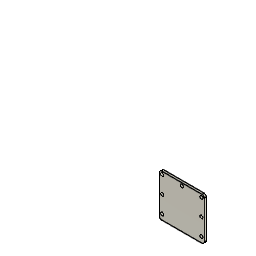
Power Panel Pro Compact - BLANK (Autodesk Fusion 360 design; units mm, degrees)
Autodesk Fusion 360 part; units mm, degrees
sketch "Sketch1" plane through (0, 175, 0) normal (0, 1, 0) x (-1, 0, 0)
  circle A0 centre (-78.5, 56) radius 1.95
  line L0 (86.5, 125) -> (-86.5, 125)
  line L1 (-86.5, 125) -> (-86.5, 0)
  line L2 (-86.5, 0) -> (86.5, 0)
  line L3 (86.5, 0) -> (86.5, 125)
  circle A1 centre (-78.5, 7.75) radius 1.95
  circle A2 centre (-23, 7.75) radius 1.95
  circle A3 centre (-11, 53.5) radius 1.95
  circle A4 centre (80.5, 53.5) radius 1.95
  circle A5 centre (80.5, 99.25) radius 1.95
  circle A6 centre (-23, 56) radius 1.95
  circle A7 centre (-50.75, 56) radius 1.95
  circle A8 centre (-78.5, 31.875) radius 1.95
  circle A9 centre (-11, 7.75) radius 1.95
  circle A10 centre (-11, 99.25) radius 1.95
  circle A11 centre (80.5, 7.75) radius 1.95
  circle A12 centre (34.75, 99.25) radius 1.95
  circle A13 centre (-23, 31.875) radius 1.95
  line L4 (-27, 3.75) -> (-74.5, 3.75)
  line L5 (-74.5, 3.75) -> (-74.5, 52)
  line L6 (-74.5, 52) -> (-27, 52)
  line L7 (-27, 52) -> (-27, 3.75)
  line L8 (76.5, 7.75) -> (-7, 7.75)
  line L9 (-7, 7.75) -> (-7, 95.25)
  line L10 (-7, 95.25) -> (76.5, 95.25)
  line L11 (76.5, 95.25) -> (76.5, 7.75)
  line L12 (-82.5, 60) -> (-19, 60)
  line L13 (-19, 60) -> (-19, 0)
  line L14 (-19, 0) -> (-82.5, 0)
  line L15 (-82.5, 0) -> (-82.5, 60)
  circle A14 centre (-78.5, 56) radius 2.15
  circle A15 centre (-50.75, 56) radius 2.15
  circle A16 centre (-23, 56) radius 2.15
  circle A17 centre (-78.5, 31.875) radius 2.15
  circle A18 centre (-23, 31.875) radius 2.15
  circle A19 centre (-78.5, 7.75) radius 2.15
  circle A20 centre (-23, 7.75) radius 2.15
  dimension "d1474" = 4
  dimension "d1475" = 4
  dimension "d1476" = 4
  dimension "d1477" = 4.3
  dimension "d1478" = 4.3
  dimension "d1479" = 4.3
  dimension "d1480" = 4.3
  dimension "d1481" = 4.3
  dimension "d1482" = 4.3
  dimension "d1483" = 4.3
  constraint horizontal L12
  constraint vertical L13
  constraint horizontal L14
  constraint vertical L15
  constraint collinear L2 L14
  constraint concentric A0 A14
  constraint concentric A7 A15
  constraint concentric A6 A16
  constraint concentric A8 A17
  constraint concentric A13 A18
  constraint concentric A1 A19
  constraint concentric A2 A20
  measures "d1474" distance of A8.centre L15
  measures "d1475" distance of A13.centre L13
  measures "d1476" distance of A7.centre L12
  measures "d1477" diameter of A14
  measures "d1478" diameter of A15
  measures "d1479" diameter of A16
  measures "d1480" diameter of A17
  measures "d1481" diameter of A18
  measures "d1482" diameter of A19
  measures "d1483" diameter of A20
extrude "Extrude1" add sketch "Sketch1" along normal blind 3 contours L2 L12 L13 L14 L15 | L4 L5 L6 L7
fillet "Fillet1" radius 3 4 edges at (19, 176.5, 0) (82.5, 176.5, 0) (82.5, 176.5, 60) (19, 176.5, 60)
equation "d1475 = d1474"
equation "d1476 = d1474"
